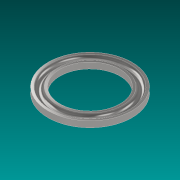
# Autodesk Inventor part: UBC Bearing 51110 - buitenkant
Saved by Autodesk Inventor 2020.2 (Build 242310000, 310)
## iProperties
Created: 2020-05-15
Part Number: UBC Bearing 51110 - buitenkant
Material: Stainless Steel
Document SubType Name: Modeling
Designer: Svend
Density: 8 g/cm^3
Appearance: Semi-Polished
Author: Svend
Autodesk Inventor part; units mm, degrees
ref_plane "YZ Plane" through (0, 0, 0) normal (1, 0, 0) x (0, 1, 0)
ref_plane "XZ Plane" through (0, 0, 0) normal (0, 1, 0) x (-1, 0, 0)
ref_plane "XY Plane" through (0, 0, 0) normal (0, 0, 1) x (1, 0, 0)
sketch "Sketch1" plane through (0, 0, 0) normal (0, 0, 1) x (1, 0, 0)
  line L0 (25, 0) -> (35, 0)
  line L1 (35, 0) -> (35, 5)
  line L2 (25, 0) -> (25, 5)
  arc A0 (27, 5) -> (33, 5) centre (30, 5) ccw
  line L3 (35, 5) -> (33, 5)
  line L4 (25, 5) -> (27, 5)
  line L5 (0, -1) -> (0, 6) projected
  point P0 (0, 0)
  point P1 (30, 0)
  dimension "d0" = 25
  dimension "d1" = 10
  dimension "d2" = 5
  dimension "d3" = 6
  constraints: 10 end point, 3 horizontal alignment, 2 horizontal, 2 point on circle, 2 vertical, 1 centre point, 1 collinear, 1 midpoint, 1 parallel, 1 vertical alignment
  measures "d0" distance of point (0, 0) L0.start
  measures "d1" distance of L0.start L0.end
  measures "d2" distance of L0.end L1.end
  measures "d3" diameter of A0
revolve "Revolution1" add sketch "Sketch1" angle 360 about axis through (0, -10, 0) along (0, 1, 0)
body "Solid1"
